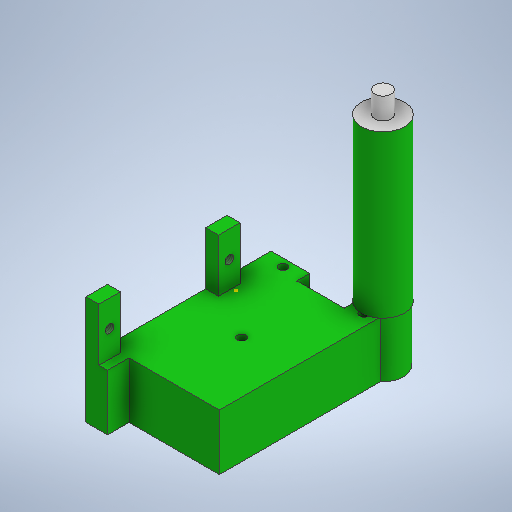
# Autodesk Inventor part: 4_2.(new).stl
Saved by Autodesk Inventor 2026.1 (Build 301233020, 233B)
## iProperties
Created: 2025-07-05
Part Number: 4_2.(new).stl
Material: Generic
Document SubType Name: Modeling
Designer: admin
Density: 1 g/cm^3
Appearance: Default
Author: admin
Autodesk Inventor part; units mm, degrees
ref_plane "YZ Plane" through (0, 0, 0) normal (1, 0, 0) x (0, 1, 0)
ref_plane "XZ Plane" through (0, 0, 0) normal (0, 1, 0) x (-1, 0, 0)
ref_plane "XY Plane" through (0, 0, 0) normal (0, 0, 1) x (1, 0, 0)
sketch "Sketch1" plane through (0, 0, 0) normal (0, 1, 0) x (-1, 0, 0)
  line L0 (4, -12.0702) -> (4, 30.9298)
  line L1 (4, 30.9298) -> (-1, 30.9298)
  line L2 (-1, 30.9298) -> (-1, 25.9298)
  line L3 (-1, 25.9298) -> (-22, 25.9298)
  line L4 (4, -12.0702) -> (-1, -12.0702)
  line L5 (-1, -12.0702) -> (-1, -12.0702)
  line L6 (-22, -8.0702) -> (-22, -8.0702)
  line L7 (-22, -8.0702) -> (-22, 3.3216)
  line L8 (-22, 3.3216) -> (-22, 3.3216)
  line L9 (-22, 3.3216) -> (-22, 25.9298)
  line L10 (-1, -12.0702) -> (-5, -12.0702)
  line L11 (-5, -12.0702) -> (-5, -9.0702)
  line L12 (-5, -9.0702) -> (-16, -9.0702)
  arc A0 (-22, -11.4735) -> (-16, -11.4735) centre (-19, -15.0915) ccw
  line L13 (-16, -9.0702) -> (-16, -11.4735)
  line L14 (-22, -8.0702) -> (-22, -11.4735)
  point P0 (0, 0)
  dimension "d28" = 5
  dimension "d30" = 0
  dimension "d69" = 5
  dimension "d118" = 4
  dimension "d119" = 3
  dimension "d130" = 4.7
  dimension "d148" = 35
  dimension "d151" = 2.4033
  constraints: 30 end point, 7 perpendicular, 2 horizontal, 2 point on circle, 2 vertical, 1 centre point, 1 parallel
  measures "d28" distance of L1.end L2.end
  measures "d30" distance of L4.end L5.end
  measures "d69" distance between parallel lines of L2 L0
  measures "d118" distance of L5.end L10.end
  measures "d119" distance of L10.end L11.end
  measures "d130" radius of A0
  measures "d148" distance between parallel lines of L3 L12
  measures "d151" distance of L12.end L13.end
extrude "Extrusion1" add sketch "Sketch1" along normal blind 13
sketch "Sketch5" plane through (0, 13, 0) normal (0, 1, 0) x (1, 0, 0)
  line L0 (-4, -30.9298) -> (1, -30.9298) projected
  line L1 (-1, -30.9298) -> (-4, -30.9298)
  line L2 (-4, -30.9298) -> (-4, -25.9298)
  line L3 (-4, -25.9298) -> (-1, -25.9298)
  line L4 (-1, -25.9298) -> (-1, -30.9298)
  line L5 (1, -30.9298) -> (1, -25.9298) projected
  line L6 (-4, 1.8702) -> (-1, 1.8702)
  line L7 (-1, 1.8702) -> (-1, -3.1298)
  line L8 (-1, -3.1298) -> (-4, -3.1298)
  line L9 (-4, -3.1298) -> (-4, 1.8702)
  line L10 (1, 12.0702) -> (1, 17.0702) projected
  line L11 (5, 12.0702) -> (-4, 12.0702) projected
  point P0 (0, 0)
  point P1 (-4, 12.0702)
  dimension "d60" = 5
  dimension "d61" = 3
  dimension "d62" = 2
  dimension "d63" = 2
  dimension "d64" = 3
  dimension "d65" = 5
  dimension "d149" = 22.8
  constraints: 16 end point, 4 parallel, 2 horizontal, 2 perpendicular, 1 point on line, 1 other
  measures "d60" distance between parallel lines of L1 L3
  measures "d61" distance between parallel lines of L4 L2
  measures "d62" distance between parallel lines of L4 L5
  measures "d63" distance between parallel lines of L7 L10
  measures "d64" distance of L7.end L8.end
  measures "d65" distance of L8.end L6.start
  measures "d149" distance between parallel lines of L8 L3
extrude "Extrusion6" add sketch "Sketch5" along normal blind 12.3
sketch "Sketch6" plane through (-1, 13, 30.9298) normal (1, 0, 0) x (0, 0, -1)
  circle A0 centre (2.5, 6.15) radius 1
  line L0 (0, 12.3) -> (5, 12.3) projected
  line L1 (0, 0) -> (0, 12.3) projected
  circle A1 centre (30.3, 6.15) radius 1
  line L2 (27.8, 12.3) -> (32.8, 12.3) projected
  line L3 (27.8, 0) -> (27.8, 12.3) projected
  point P0 (30.9298, -13)
  dimension "d70" = 2
  dimension "d71" = 6.15
  dimension "d72" = 2.5
  dimension "d73" = 2
  dimension "d74" = 6.15
  dimension "d75" = 2.5
  constraints: 2 centre point
  measures "d70" diameter of A0
  measures "d71" distance from line of A0.centre L0
  measures "d72" distance from line of L1 A0.centre
  measures "d73" diameter of A1
  measures "d74" distance from line of A1.centre L2
  measures "d75" distance from line of A1.centre L3
extrude "Extrusion7" cut sketch "Sketch6" against normal blind 12.3
thread "Thread6" size "M2x0.4" class "6H" standard "ANSI Metric M Profile" length 10
thread "Thread7" size "M2x0.4" class "6H" standard "ANSI Metric M Profile" length 10
sketch "Sketch10" plane through (0, 13, 0) normal (0, 1, 0) x (1, 0, 0)
  circle A0 centre (0.6, 10.2702) radius 1
  circle A1 centre (19.4, 10.2702) radius 1
  circle A2 centre (10, -8.7298) radius 1
  line L0 (1, -25.9298) -> (22, -25.9298) projected
  line L1 (-4, -3.1298) -> (-4, -25.9298) projected
  line L2 (5, 12.0702) -> (-4, 12.0702) projected
  line L3 (5, 9.0702) -> (5, 12.0702) projected
  line L4 (5, 12.0702) -> (1, 12.0702) projected
  point P0 (0, 0)
  point P1 (1, 17.0702)
  point P2 (-1, 17.0702)
  point P3 (-4, 12.0702)
  dimension "d108" = 2
  dimension "d109" = 2
  dimension "d110" = 2
  dimension "d111" = 9.4
  dimension "d112" = 9.4
  dimension "d113" = 19
  dimension "d117" = 19
  dimension "d121" = 14
  dimension "d150" = 1.8
  constraints: 3 centre point, 1 other
  measures "d108" diameter of A0
  measures "d109" diameter of A1
  measures "d110" diameter of A2
  measures "d111" horizontal distance of A0.centre A2.centre
  measures "d112" horizontal distance of A2.centre A1.centre
  measures "d113" vertical distance of A2.centre A1.centre
  measures "d117" vertical distance of A2.centre A0.centre
  measures "d121" distance from line of L1 A2.centre
  measures "d150" distance from line of A0.centre L4
extrude "Extrusion11" cut sketch "Sketch10" against normal blind 15
sketch "Sketch13" plane through (0, 13, 0) normal (0, 1, 0) x (1, 0, 0)
  point P0 (0, 0)
sketch "Sketch14" plane through (0, 0, 0) normal (0, -1, 0) x (1, 0, 0)
  circle A0 centre (19.4611, -14.5702) radius 2
  circle A1 centre (19.4, -10.2702) radius 1 projected
  point P0 (0, 0)
  dimension "d131" = 4
  dimension "d132" = 4.3
  constraints: 1 centre point
  measures "d131" diameter of A0
  measures "d132" vertical distance of A0.centre A1.centre
extrude "Extrusion12" cut sketch "Sketch14" against normal blind 6 contours A0
sketch "Sketch15" plane through (0, 13, 0) normal (0, 1, 0) x (1, 0, 0)
  arc A0 (22, 11.4735) -> (16, 11.4735) centre (19, 15.0915) ccw projected
  line L0 (15.3998, 12.0702) -> (22.6002, 12.0702)
  arc A1 (22.6002, 12.0702) -> (15.3998, 12.0702) centre (19, 15.0915) ccw
  line L1 (1, -25.9298) -> (22, -25.9298) projected
  point P0 (0, 0)
  dimension "d135" = 22.8
  constraints: 4 point on circle, 2 end point, 1 centre point, 1 horizontal
extrude "Extrusion13" add sketch "Sketch15" along normal blind 12.5
sketch "Sketch16" plane through (0, 25.5, 0) normal (0, 1, 0) x (1, 0, 0)
  arc A0 (22, 11.4735) -> (16, 11.4735) centre (19, 15.0915) ccw projected
  circle A1 centre (19, 15.0915) radius 5
  point P0 (0, 0)
  dimension "d138" = 10
  constraints: 1 centre point, 1 coincident
  measures "d138" diameter of A1
extrude "Extrusion14" add sketch "Sketch16" along normal mid plane 25
sketch "Sketch18" plane through (19, 38, -15.0915) normal (0, 1, 0) x (1, 0, 0)
  circle A0 centre (0, 0) radius 5
  point P0 (-19, -15.0915)
  constraints: 1 centre point
extrude "Extrusion16" add sketch "Sketch18" along normal blind 12.5
sketch "Sketch19" plane through (19, 50.5, -15.0915) normal (0, 1, 0) x (1, 0, 0)
  circle A0 centre (0, 0) radius 1.9
  point P0 (-19, -15.0915)
  dimension "d154" = 3.8
  constraints: 1 centre point
  measures "d154" diameter of A0
extrude "Extrusion17" add sketch "Sketch19" along normal blind 5
body "Solid1"
